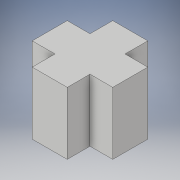
# Autodesk Inventor part: vertibrae to pelvis connector
Saved by Autodesk Inventor 2019.3 (Build 233278000, 278)
## iProperties
Created: 2018-12-20
Part Number: vertibrae to pelvis connector
Material: Generic
Document SubType Name: Modeling
Designer: Frienddo
Density: 1 g/cm^3
Appearance: Default
Author: Frienddo
Autodesk Inventor part; units mm, degrees
ref_plane "YZ Plane" through (0, 0, 0) normal (1, 0, 0) x (0, 1, 0)
ref_plane "XZ Plane" through (0, 0, 0) normal (0, 1, 0) x (-1, 0, 0)
ref_plane "XY Plane" through (0, 0, 0) normal (0, 0, 1) x (1, 0, 0)
sketch "Sketch1" plane through (0, 0, 0) normal (0, 1, 0) x (-1, 0, 0)
  line L0 (0, 0) -> (6.455, 0)
  line L1 (6.455, 0) -> (6.455, 2.8076)
  line L2 (6.455, 2.8076) -> (2.8076, 2.8076)
  line L3 (2.8076, 2.8076) -> (2.8076, 6.455)
  line L4 (2.8076, 6.455) -> (0, 6.455)
  line L5 (0, 6.455) -> (0, 0)
  line L6 (0, 6.455) -> (-2.8076, 6.455)
  line L7 (-2.8076, 6.455) -> (-2.8076, 2.8076)
  line L8 (-2.8076, 2.8076) -> (-6.455, 2.8076)
  line L9 (-6.455, 2.8076) -> (-6.455, 0)
  line L10 (-6.455, 0) -> (0, 0)
  line L11 (0, 0) -> (0, 6.455)
  line L12 (-6.455, 0) -> (-6.455, -2.8076)
  line L13 (-6.455, -2.8076) -> (-2.8076, -2.8076)
  line L14 (-2.8076, -2.8076) -> (-2.8076, -6.455)
  line L15 (-2.8076, -6.455) -> (0, -6.455)
  line L16 (0, -6.455) -> (0, 0)
  line L17 (0, 0) -> (-6.455, 0)
  line L18 (0, -6.455) -> (2.8076, -6.455)
  line L19 (2.8076, -6.455) -> (2.8076, -2.8076)
  line L20 (2.8076, -2.8076) -> (6.455, -2.8076)
  line L21 (6.455, -2.8076) -> (6.455, 0)
  line L22 (6.455, 0) -> (0, 0)
  line L23 (0, 0) -> (0, -6.455)
  dimension "d2" = 360
  constraints: 48 end point, 7 perpendicular, 2 coincident, 1 horizontal, 47 other
extrude "Extrusion1" add sketch "Sketch1" along normal blind 10
body "Solid1"
